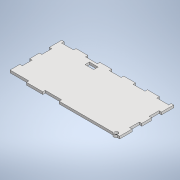
# Autodesk Inventor part: Wall 1
Saved by Autodesk Inventor 2020 (Build 240168000, 168)
## iProperties
Created: 2022-02-16
Part Number: Wall 1
Material: Generic
Document SubType Name: Modeling
Designer: rwte
Density: 1 g/cm^3
Appearance: Default
Author: rwte
Autodesk Inventor part; units mm, degrees
ref_plane "YZ Plane" through (0, 0, 0) normal (1, 0, 0) x (0, 1, 0)
ref_plane "XZ Plane" through (0, 0, 0) normal (0, 1, 0) x (-1, 0, 0)
ref_plane "XY Plane" through (0, 0, 0) normal (0, 0, 1) x (1, 0, 0)
sketch "Sketch1" plane through (0, 0, 0) normal (0, 1, 0) x (-1, 0, 0)
  line L0 (-65.5, -30) -> (65.5, -30)
  line L1 (65.5, -30) -> (65.5, 30)
  line L2 (65.5, 30) -> (-65.5, 30)
  line L3 (-65.5, 30) -> (-65.5, -30)
  line L4 (-65.5, -30) -> (65.5, 30) construction
  line L5 (65.5, -30) -> (-65.5, 30) construction
  line L6 (-65.5, 30) -> (-65.5, 18)
  line L7 (-65.5, 18) -> (-68.5, 18)
  line L8 (-68.5, 18) -> (-68.5, 30)
  line L9 (-68.5, 30) -> (-65.5, 30)
  line L10 (-65.5, -30) -> (-65.5, -18)
  line L11 (-65.5, -18) -> (-68.5, -18)
  line L12 (-68.5, -18) -> (-68.5, -30)
  line L13 (-68.5, -30) -> (-65.5, -30)
  line L14 (65.5, -30) -> (50.9444, -30)
  line L15 (50.9444, -30) -> (50.9444, -33)
  line L16 (50.9444, -33) -> (65.5, -33)
  line L17 (65.5, -33) -> (65.5, -30)
  line L18 (-65.5, -30) -> (-50.9444, -30)
  line L19 (-50.9444, -30) -> (-50.9444, -33)
  line L20 (-50.9444, -33) -> (-65.5, -33)
  line L21 (-65.5, -33) -> (-65.5, -30)
  line L22 (-65.5, 6) -> (-65.5, -6)
  line L23 (-65.5, -6) -> (-68.5, -6)
  line L24 (-68.5, -6) -> (-68.5, 6)
  line L25 (-68.5, 6) -> (-65.5, 6)
  line L26 (-21.8333, -30) -> (-36.3889, -30)
  line L27 (-36.3889, -30) -> (-36.3889, -33)
  line L28 (-36.3889, -33) -> (-21.8333, -33)
  line L29 (-21.8333, -33) -> (-21.8333, -30)
  line L30 (7.2778, -30) -> (-7.2778, -30)
  line L31 (-7.2778, -30) -> (-7.2778, -33)
  line L32 (-7.2778, -33) -> (7.2778, -33)
  line L33 (7.2778, -33) -> (7.2778, -30)
  line L34 (36.3889, -30) -> (21.8333, -30)
  line L35 (21.8333, -30) -> (21.8333, -33)
  line L36 (21.8333, -33) -> (36.3889, -33)
  line L37 (36.3889, -33) -> (36.3889, -30)
  line L38 (0, -46.5854) -> (0, 48.5125) projected
  line L39 (88.9, 0) -> (-88.9, 0) projected
  line L40 (65.5, 30) -> (65.5, -30)
  line L41 (65.5, 30) -> (65.5, 18)
  line L42 (65.5, 18) -> (68.5, 18)
  line L43 (68.5, 18) -> (68.5, 30)
  line L44 (68.5, 30) -> (65.5, 30)
  line L45 (65.5, -30) -> (65.5, -18)
  line L46 (65.5, -18) -> (68.5, -18)
  line L47 (68.5, -18) -> (68.5, -30)
  line L48 (68.5, -30) -> (65.5, -30)
  line L49 (65.5, -33) -> (65.5, -30)
  line L50 (65.5, 6) -> (65.5, -6)
  line L51 (65.5, -6) -> (68.5, -6)
  line L52 (68.5, -6) -> (68.5, 6)
  line L53 (68.5, 6) -> (65.5, 6)
  line L54 (50.9444, 30) -> (50.9444, 33)
  line L55 (50.9444, 33) -> (65.5, 33)
  line L56 (65.5, 33) -> (65.5, 30)
  line L57 (-50.9444, 30) -> (-50.9444, 33)
  line L58 (-50.9444, 33) -> (-65.5, 33)
  line L59 (-65.5, 33) -> (-65.5, 30)
  line L60 (-36.3889, 30) -> (-36.3889, 33)
  line L61 (-36.3889, 33) -> (-21.8333, 33)
  line L62 (-21.8333, 33) -> (-21.8333, 30)
  line L63 (-7.2778, 30) -> (-7.2778, 33)
  line L64 (-7.2778, 33) -> (7.2778, 33)
  line L65 (7.2778, 33) -> (7.2778, 30)
  line L66 (21.8333, 30) -> (21.8333, 33)
  line L67 (21.8333, 33) -> (36.3889, 33)
  line L68 (36.3889, 33) -> (36.3889, 30)
  line L69 (68.5, -33) -> (-68.5, -33)
  line L70 (-68.5, -33) -> (-68.5, 33)
  line L71 (-68.5, 33) -> (68.5, 33)
  line L72 (68.5, 33) -> (68.5, -33)
  line L73 (68.5, -33) -> (-68.5, 33) construction
  line L74 (-68.5, -33) -> (68.5, 33) construction
  point P0 (0, 0)
  point P1 (58.2222, -33)
  point P2 (-58.2222, -33)
  point P3 (-68.5, -24)
  point P4 (-68.5, 24)
  point P5 (-68.5, 0)
  point P6 (0, -33)
  point P7 (0, -30)
  point P8 (29.1111, -33)
  point P9 (-29.1111, -33)
  point P10 (68.5, -24)
  point P11 (68.5, 24)
  point P12 (68.5, 0)
  point P13 (-7.2778, -33)
  point P14 (7.2778, -33)
  point P15 (21.8333, -33)
  point P16 (36.3889, -33)
  dimension "d0" = 131
  dimension "d1" = 60
  dimension "d2" = 12
  dimension "d3" = 14.5556
  dimension "d4" = 14.5556
  dimension "d5" = 3
  dimension "d6" = 12
  dimension "d7" = 12
  dimension "d8" = 12
  dimension "d9" = 14.5556
  dimension "d10" = 14.5556
  dimension "d11" = 14.5556
  dimension "d12" = 14.5556
  dimension "d13" = 14.5556
  dimension "d14" = 14.5556
  constraints: 144 end point, 31 symmetric about line, 20 parallel, 13 midpoint, 10 perpendicular, 8 point on line, 5 horizontal alignment, 4 vertical alignment, 1 horizontal, 1 vertical, 11 other
  measures "d0" distance of L1.end L2.end
  measures "d1" distance of L2.end L3.end
  measures "d2" distance of L8.end L7.end
  measures "d3" distance of L20.end L19.end
  measures "d4" distance of L16.end L15.end
  measures "d5" distance of L2.end L8.end
  measures "d6" distance of L11.end L12.end
  measures "d7" distance of L23.end L24.end
  measures "d8" distance of L24.end L7.end
  measures "d9" distance of L19.end L27.end
  measures "d10" distance of L28.end L31.end
  measures "d11" distance of L35.end L32.end
  measures "d12" distance of L27.end L28.end
  measures "d13" distance of L35.end L36.end
  measures "d14" distance of L15.end L36.end
extrude "Extrusion1" add sketch "Sketch1" along normal blind 3 contours L3 L39 L38 L0 | L13 L12 L11 L3 | L21 L69 L70 L13 | L0 L27 L69 L19 | L23 L24 L39 L3 | L0 L31 L69 L29 | L39 L24 L25 L3 | L3 L2 L38 L39 | L39 L1 L0 L38 | L38 L2 L1 L39 | L7 L8 L9 L3 | L39 L52 L51 L1 | L1 L53 L52 L39 | L0 L35 L69 L33 | L46 L47 L48 L1 | L1 L44 L43 L42 | L0 L15 L69 L37 | L48 L72 L69 L17
sketch "Sketch5" plane through (0, 0, 0) normal (0, -1, 0) x (1, 0, 0)
  line L0 (68.5, 30) -> (68.5, 18) projected
  line L1 (-68.5, 30) -> (68.5, 30) projected
  line L2 (-68.5, 18) -> (-68.5, 30) projected
  line L3 (-65.5, 18) -> (-68.5, 18) projected
  line L4 (-65.5, 6) -> (-65.5, 18) projected
  line L5 (-68.5, 6) -> (-65.5, 6) projected
  line L6 (-68.5, -6) -> (-68.5, 6) projected
  line L7 (-65.5, -6) -> (-68.5, -6) projected
  line L8 (-65.5, -18) -> (-65.5, -6) projected
  line L9 (-68.5, -18) -> (-65.5, -18) projected
  line L10 (-68.5, -33) -> (-68.5, -18) projected
  line L11 (-65.5, -33) -> (-68.5, -33) projected
  line L12 (-65.5, -30) -> (-65.5, -33) projected
  line L13 (-50.9444, -30) -> (-65.5, -30) projected
  line L14 (-50.9444, -33) -> (-50.9444, -30) projected
  line L15 (-36.3889, -33) -> (-50.9444, -33) projected
  line L16 (-36.3889, -30) -> (-36.3889, -33) projected
  line L17 (-21.8333, -30) -> (-36.3889, -30) projected
  line L18 (-21.8333, -33) -> (-21.8333, -30) projected
  line L19 (-7.2778, -33) -> (-21.8333, -33) projected
  line L20 (-7.2778, -30) -> (-7.2778, -33) projected
  line L21 (7.2778, -30) -> (-7.2778, -30) projected
  line L22 (7.2778, -33) -> (7.2778, -30) projected
  line L23 (21.8333, -33) -> (7.2778, -33) projected
  line L24 (21.8333, -30) -> (21.8333, -33) projected
  line L25 (36.3889, -30) -> (21.8333, -30) projected
  line L26 (36.3889, -33) -> (36.3889, -30) projected
  line L27 (50.9444, -33) -> (36.3889, -33) projected
  line L28 (50.9444, -30) -> (50.9444, -33) projected
  line L29 (65.5, -30) -> (50.9444, -30) projected
  line L30 (65.5, -33) -> (65.5, -30) projected
  line L31 (68.5, -33) -> (65.5, -33) projected
  line L32 (68.5, -18) -> (68.5, -33) projected
  line L33 (65.5, -18) -> (68.5, -18) projected
  line L34 (65.5, -6) -> (65.5, -18) projected
  line L35 (68.5, -6) -> (65.5, -6) projected
  line L36 (68.5, 6) -> (68.5, -6) projected
  line L37 (65.5, 6) -> (68.5, 6) projected
  line L38 (65.5, 18) -> (65.5, 6) projected
  line L39 (68.5, 18) -> (65.5, 18) projected
  line L40 (-45.5, 30) -> (-25.5, 30)
  line L41 (-25.5, 30) -> (-25.5, 33)
  line L42 (-25.5, 33) -> (-45.5, 33)
  line L43 (-45.5, 33) -> (-45.5, 30)
  point P0 (0, 0)
  point P1 (-35.5, 33)
  dimension "d26" = 20
  dimension "d27" = 23
  constraints: 8 end point, 2 parallel, 2 point on line, 1 midpoint, 1 perpendicular
  measures "d26" distance of L41.end L42.end
  measures "d27" distance of L1.start L40.start
extrude "Extrusion5" add sketch "Sketch5" against normal up to surface (3 mm away) contours L1 L43 L42 L41
sketch "Sketch6" plane through (0, 0, 0) normal (0, -1, 0) x (1, 0, 0)
  line L0 (-68.5, 30) -> (-45.5, 30) projected
  line L1 (-68.5, 18) -> (-68.5, 30) projected
  line L2 (-65.5, 18) -> (-68.5, 18) projected
  line L3 (-65.5, 6) -> (-65.5, 18) projected
  line L4 (-68.5, 6) -> (-65.5, 6) projected
  line L5 (-68.5, -6) -> (-68.5, 6) projected
  line L6 (-65.5, -6) -> (-68.5, -6) projected
  line L7 (-65.5, -18) -> (-65.5, -6) projected
  line L8 (-68.5, -18) -> (-65.5, -18) projected
  line L9 (-68.5, -33) -> (-68.5, -18) projected
  line L10 (-65.5, -33) -> (-68.5, -33) projected
  line L11 (-65.5, -30) -> (-65.5, -33) projected
  line L12 (-50.9444, -30) -> (-65.5, -30) projected
  line L13 (-50.9444, -33) -> (-50.9444, -30) projected
  line L14 (-36.3889, -33) -> (-50.9444, -33) projected
  line L15 (-36.3889, -30) -> (-36.3889, -33) projected
  line L16 (-21.8333, -30) -> (-36.3889, -30) projected
  line L17 (-21.8333, -33) -> (-21.8333, -30) projected
  line L18 (-7.2778, -33) -> (-21.8333, -33) projected
  line L19 (-7.2778, -30) -> (-7.2778, -33) projected
  line L20 (7.2778, -30) -> (-7.2778, -30) projected
  line L21 (7.2778, -33) -> (7.2778, -30) projected
  line L22 (21.8333, -33) -> (7.2778, -33) projected
  line L23 (21.8333, -30) -> (21.8333, -33) projected
  line L24 (36.3889, -30) -> (21.8333, -30) projected
  line L25 (36.3889, -33) -> (36.3889, -30) projected
  line L26 (50.9444, -33) -> (36.3889, -33) projected
  line L27 (50.9444, -30) -> (50.9444, -33) projected
  line L28 (65.5, -30) -> (50.9444, -30) projected
  line L29 (65.5, -33) -> (65.5, -30) projected
  line L30 (68.5, -33) -> (65.5, -33) projected
  line L31 (68.5, -18) -> (68.5, -33) projected
  line L32 (65.5, -18) -> (68.5, -18) projected
  line L33 (65.5, -6) -> (65.5, -18) projected
  line L34 (68.5, -6) -> (65.5, -6) projected
  line L35 (68.5, 6) -> (68.5, -6) projected
  line L36 (65.5, 6) -> (68.5, 6) projected
  line L37 (65.5, 18) -> (65.5, 6) projected
  line L38 (68.5, 18) -> (65.5, 18) projected
  line L39 (68.5, 30) -> (68.5, 18) projected
  line L40 (-25.5, 30) -> (68.5, 30) projected
  line L41 (-25.5, 30) -> (-25.5, 33) projected
  line L42 (-25.5, 33) -> (-45.5, 33) projected
  line L43 (-45.5, 33) -> (-45.5, 30) projected
  line L44 (-25.5, 30) -> (68.5, 30) projected
  line L45 (-5.5, 30) -> (64.5, 30)
  line L46 (64.5, 30) -> (64.5, 33)
  line L47 (64.5, 33) -> (-5.5, 33)
  line L48 (-5.5, 33) -> (-5.5, 30)
  line L49 (61.5, 33) -> (61.5, 30)
  line L50 (64.5, 31.5) -> (61.5, 31.5) construction
  circle A0 centre (63, 31.6771) radius 2.25
  circle A1 centre (63, 31.6771) radius 4
  line L51 (64.82, 33) -> (68.5, 33)
  line L52 (68.5, 30) -> (68.5, 18) projected
  line L53 (68.5, 30) -> (68.5, 33)
  point P0 (0, 0)
  point P1 (59.2251, 33)
  point P2 (59.3685, 30)
  point P3 (66.6315, 30)
  point P4 (66.7749, 33)
  dimension "d30" = 70
  dimension "d31" = 20
  dimension "d32" = 3
  dimension "d33" = 4.5
  dimension "d34" = 8
  constraints: 16 end point, 3 point on circle, 3 point on line, 2 centre point, 2 horizontal, 2 horizontal alignment, 2 midpoint, 2 parallel, 2 vertical, 1 coincident, 1 perpendicular
  measures "d30" distance of L46.end L47.end
  measures "d31" distance of L41.end L47.end
  measures "d32" distance between parallel lines of L49 L46
  measures "d33" diameter of A0
  measures "d34" diameter of A1
extrude "Extrusion6" add sketch "Sketch6" against normal blind 3 contours L48 L47 A1 L40 | A1 L47 A0 L40 | L40 A0 A1 | A1 L51 A0 L47 | A1 L51 L53 L40 | L40 A0 L51 A1
sketch "Sketch7" plane through (0, 0, 0) normal (0, -1, 0) x (1, 0, 0)
  line L0 (-25.5, 30) -> (-5.5, 30) projected
  line L1 (-25.5, 30) -> (-25.5, 33) projected
  line L2 (-25.5, 33) -> (-45.5, 33) projected
  line L3 (-45.5, 33) -> (-45.5, 30) projected
  line L4 (-68.5, 30) -> (-45.5, 30) projected
  line L5 (-68.5, 18) -> (-68.5, 30) projected
  line L6 (-65.5, 18) -> (-68.5, 18) projected
  line L7 (-65.5, 6) -> (-65.5, 18) projected
  line L8 (-68.5, 6) -> (-65.5, 6) projected
  line L9 (-68.5, -6) -> (-68.5, 6) projected
  line L10 (-65.5, -6) -> (-68.5, -6) projected
  line L11 (-65.5, -18) -> (-65.5, -6) projected
  line L12 (-68.5, -18) -> (-65.5, -18) projected
  line L13 (-68.5, -33) -> (-68.5, -18) projected
  line L14 (-65.5, -33) -> (-68.5, -33) projected
  line L15 (-65.5, -30) -> (-65.5, -33) projected
  line L16 (-50.9444, -30) -> (-65.5, -30) projected
  line L17 (-50.9444, -33) -> (-50.9444, -30) projected
  line L18 (-36.3889, -33) -> (-50.9444, -33) projected
  line L19 (-36.3889, -30) -> (-36.3889, -33) projected
  line L20 (-21.8333, -30) -> (-36.3889, -30) projected
  line L21 (-21.8333, -33) -> (-21.8333, -30) projected
  line L22 (-7.2778, -33) -> (-21.8333, -33) projected
  line L23 (-7.2778, -30) -> (-7.2778, -33) projected
  line L24 (7.2778, -30) -> (-7.2778, -30) projected
  line L25 (7.2778, -33) -> (7.2778, -30) projected
  line L26 (21.8333, -33) -> (7.2778, -33) projected
  line L27 (21.8333, -30) -> (21.8333, -33) projected
  line L28 (36.3889, -30) -> (21.8333, -30) projected
  line L29 (36.3889, -33) -> (36.3889, -30) projected
  line L30 (50.9444, -33) -> (36.3889, -33) projected
  line L31 (50.9444, -30) -> (50.9444, -33) projected
  line L32 (65.5, -30) -> (50.9444, -30) projected
  line L33 (65.5, -33) -> (65.5, -30) projected
  line L34 (68.5, -33) -> (65.5, -33) projected
  line L35 (68.5, -18) -> (68.5, -33) projected
  line L36 (65.5, -18) -> (68.5, -18) projected
  line L37 (65.5, -6) -> (65.5, -18) projected
  line L38 (68.5, -6) -> (65.5, -6) projected
  line L39 (68.5, 6) -> (68.5, -6) projected
  line L40 (65.5, 6) -> (68.5, 6) projected
  line L41 (65.5, 18) -> (65.5, 6) projected
  line L42 (68.5, 18) -> (65.5, 18) projected
  line L43 (68.5, 18) -> (68.5, 33) projected
  line L44 (68.5, 33) -> (66.7749, 33) projected
  arc A0 (66.7749, 33) -> (59.2251, 33) centre (63, 31.6771) ccw projected
  line L45 (59.2251, 33) -> (-5.5, 33) projected
  line L46 (-5.5, 33) -> (-5.5, 30) projected
  arc A1 (64.5, 30) -> (61.5, 30) centre (63, 31.6771) ccw projected
  line L47 (61.5, 30) -> (64.5, 30) projected
  circle A2 centre (63, 31.6771) radius 2.25
  point P0 (0, 0)
  constraints: 1 centre point, 1 coincident, 1 concentric
extrude "Extrusion7" cut sketch "Sketch7" against normal blind 3 contours A2 L47
sketch "Sketch8" plane through (0, 3, 0) normal (0, 1, 0) x (1, 0, 0)
  line L0 (-5.5, -30) -> (-5.5, -33) projected
  line L1 (-5.5, -33) -> (59.2251, -33) projected
  arc A0 (59.2251, -33) -> (66.7749, -33) centre (63, -31.6771) ccw projected
  line L2 (66.7749, -33) -> (68.5, -33) projected
  line L3 (68.5, -33) -> (68.5, -18) projected
  line L4 (68.5, -18) -> (65.5, -18) projected
  line L5 (65.5, -18) -> (65.5, -6) projected
  line L6 (65.5, -6) -> (68.5, -6) projected
  line L7 (68.5, -6) -> (68.5, 6) projected
  line L8 (68.5, 6) -> (65.5, 6) projected
  line L9 (65.5, 6) -> (65.5, 18) projected
  line L10 (65.5, 18) -> (68.5, 18) projected
  line L11 (68.5, 18) -> (68.5, 33) projected
  line L12 (68.5, 33) -> (65.5, 33) projected
  line L13 (65.5, 33) -> (65.5, 30) projected
  line L14 (65.5, 30) -> (50.9444, 30) projected
  line L15 (50.9444, 30) -> (50.9444, 33) projected
  line L16 (50.9444, 33) -> (36.3889, 33) projected
  line L17 (36.3889, 33) -> (36.3889, 30) projected
  line L18 (36.3889, 30) -> (21.8333, 30) projected
  line L19 (21.8333, 30) -> (21.8333, 33) projected
  line L20 (21.8333, 33) -> (7.2778, 33) projected
  line L21 (7.2778, 33) -> (7.2778, 30) projected
  line L22 (7.2778, 30) -> (-7.2778, 30) projected
  line L23 (-7.2778, 30) -> (-7.2778, 33) projected
  line L24 (-7.2778, 33) -> (-21.8333, 33) projected
  line L25 (-21.8333, 33) -> (-21.8333, 30) projected
  line L26 (-21.8333, 30) -> (-36.3889, 30) projected
  line L27 (-36.3889, 30) -> (-36.3889, 33) projected
  line L28 (-36.3889, 33) -> (-50.9444, 33) projected
  line L29 (-50.9444, 33) -> (-50.9444, 30) projected
  line L30 (-50.9444, 30) -> (-65.5, 30) projected
  line L31 (-65.5, 30) -> (-65.5, 33) projected
  line L32 (-65.5, 33) -> (-68.5, 33) projected
  line L33 (-68.5, 33) -> (-68.5, 18) projected
  line L34 (-68.5, 18) -> (-65.5, 18) projected
  line L35 (-65.5, 18) -> (-65.5, 6) projected
  line L36 (-65.5, 6) -> (-68.5, 6) projected
  line L37 (-68.5, 6) -> (-68.5, -6) projected
  line L38 (-68.5, -6) -> (-65.5, -6) projected
  line L39 (-65.5, -6) -> (-65.5, -18) projected
  line L40 (-65.5, -18) -> (-68.5, -18) projected
  line L41 (-68.5, -18) -> (-68.5, -30) projected
  line L42 (-68.5, -30) -> (-45.5, -30) projected
  line L43 (-45.5, -33) -> (-45.5, -30) projected
  line L44 (-25.5, -33) -> (-45.5, -33) projected
  line L45 (-25.5, -30) -> (-25.5, -33) projected
  line L46 (-25.5, -30) -> (-5.5, -30) projected
  circle A1 centre (63, -31.6771) radius 2.25 projected
  line L47 (-17.9, 21.5) -> (-28.5, 21.5)
  line L48 (-28.5, 21.5) -> (-28.5, 27)
  line L49 (-28.5, 27) -> (-17.9, 27)
  line L50 (-17.9, 27) -> (-17.9, 21.5)
  point P0 (0, 0)
  dimension "d41" = 10.6
  dimension "d42" = 5.5
  dimension "d45" = 40
  dimension "d46" = 3
  constraints: 8 end point, 2 parallel, 1 horizontal, 1 perpendicular
  measures "d41" distance of L47.start L47.end
  measures "d42" distance of L47.end L48.end
  measures "d45" distance between parallel lines of L33 L48
  measures "d46" distance between parallel lines of L26 L49
extrude "Extrusion8" cut sketch "Sketch8" against normal through all contours L47 L48 L49 L50
equation "\"d2\" = 0.2 * d1"
equation "\"d3\" = 0.111111 * d0"
equation "\"d4\" = d3"
equation "\"d6\" = d2"
equation "\"d7\" = d2"
equation "\"d8\" = d2"
equation "\"d9\" = d3"
equation "\"d10\" = d9"
equation "\"d11\" = d10"
equation "\"d12\" = d9"
equation "\"d13\" = d3"
equation "\"d14\" = d3"
equation "\"d15\" = d5"
body "Solid1"
